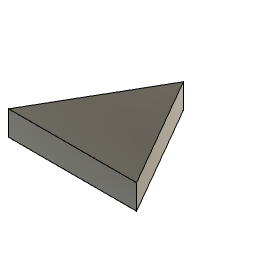
Test3 (Autodesk Fusion 360 design; units mm, degrees)
Autodesk Fusion 360 part; units mm, degrees
sketch "Sketch1" plane through (0, 0, 0) normal (0, 0, 1) x (1, 0, 0)
  line L0 (0, 30) -> (-25.9808, -15)
  line L1 (-25.9808, -15) -> (25.9808, -15)
  line L2 (25.9808, -15) -> (0, 30)
  dimension "d1" = 30
  measures "d1" distance of L0.start origin
extrude "Extrude1" add sketch "Sketch1" along normal blind 10
